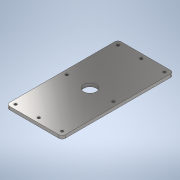
# Autodesk Inventor part: МПСТ люк
Saved by Autodesk Inventor 2022.1 (Build 261234020, 234B)
## iProperties
Created: 2021-12-13
Part Number: МПСТ люк
Material: Сталь, углеродистая
Document SubType Name: Modeling
Designer: Алексанян Г.
Density: 7.85 g/cm^3
Appearance: С умеренной полировкой
Author: Алексанян Г.
Autodesk Inventor part; units mm, degrees
ref_plane "YZ Plane" through (0, 0, 0) normal (1, 0, 0) x (0, 1, 0)
ref_plane "XZ Plane" through (0, 0, 0) normal (0, 1, 0) x (-1, 0, 0)
ref_plane "XY Plane" through (0, 0, 0) normal (0, 0, 1) x (1, 0, 0)
sketch "Эскиз1" plane through (0, 0, 0) normal (0, 1, 0) x (-1, 0, 0)
  line L0 (90, -180) -> (-90, -180)
  line L1 (-90, -180) -> (-90, 180)
  line L2 (-90, 180) -> (90, 180)
  line L3 (90, 180) -> (90, -180)
  line L4 (90, -180) -> (-90, 180) construction
  line L5 (-90, -180) -> (90, 180) construction
  point P0 (0, 0)
  dimension "d0" = 180
  dimension "d1" = 360
  constraints: 12 end point, 2 midpoint, 2 parallel, 1 horizontal, 1 perpendicular
  measures "d0" distance of L1.end L2.end
  measures "d1" distance of L0.end L1.end
extrude "Выдавливание1" add sketch "Эскиз1" along normal blind 10
fillet "Сопряжение1" radius 10 4 edges at (-90, 5, -180) (-90, 5, 180) (90, 5, 180) (90, 5, -180)
sketch "Эскиз2" plane through (0, 10, 0) normal (0, 1, 0) x (1, 0, 0)
  line L0 (90, -170) -> (90, 170) projected
  line L1 (-80, -180) -> (80, -180) projected
  line L2 (0, 185.9906) -> (0, -228.4226) construction
  line L3 (-161.892, 0) -> (248.2378, 0) construction
  point P0 (0, 0)
  point P1 (75, -165)
  point P2 (75, 0)
  point P3 (0, -165)
  point P4 (75, 165)
  point P5 (0, 165)
  point P6 (-75, -165)
  point P7 (-75, 0)
  point P8 (-75, 165)
  point P9 (90, 0)
  dimension "d5" = 15
  dimension "d7" = 15
  constraints: 5 symmetric about line, 4 end point, 3 horizontal alignment, 3 vertical alignment, 1 horizontal, 1 midpoint, 1 vertical
  measures "d5" distance from line of L0 point (75, 0)
  measures "d7" distance from line of L1 point (75, -165)
hole "Отверстие1" at (75, 10, 165) at (75, 10, 0) at (0, 10, 165) at (0, 10, -165) at (75, 10, -165) at (-75, 10, -165) at (-75, 10, 0) at (-75, 10, 165) direction (0, -1, 0) diameter 8.376 end through all thread size "M10x1.5" class "6H" standard "ISO Metric profile"
sketch "Эскиз3" plane through (0, 10, 0) normal (0, 1, 0) x (1, 0, 0)
  circle A0 centre (0, 0) radius 20
  dimension "d15" = 40
  constraints: 1 centre point, 1 coincident
  measures "d15" diameter of A0
extrude "Выдавливание2" cut sketch "Эскиз3" against normal through all
